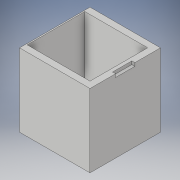
# Autodesk Inventor part: Base1
Saved by Autodesk Inventor 2017 (Build 210142000, 142)
## iProperties
Created: 2018-12-22
Part Number: Base1
Material: Generic
Document SubType Name: Modeling
Designer: Cj Lohnes
Density: 1 g/cm^3
Appearance: Default
Mass: 460.828 g
Surface Area: 957.236 cm^2
Volume: 460.828 cm^3
Author: Cj Lohnes
Autodesk Inventor part; units mm, degrees
ref_plane "YZ Plane" through (0, 0, 0) normal (1, 0, 0) x (0, 1, 0)
ref_plane "XZ Plane" through (0, 0, 0) normal (0, 1, 0) x (-1, 0, 0)
ref_plane "XY Plane" through (0, 0, 0) normal (0, 0, 1) x (1, 0, 0)
sketch "Sketch1" plane through (0, 0, 0) normal (0, 1, 0) x (-1, 0, 0)
  line L0 (66.3492, 132.9478) -> (-43.6508, 132.9478)
  line L1 (-43.6508, 132.9478) -> (-43.6508, 22.9478)
  line L2 (-43.6508, 22.9478) -> (66.3492, 22.9478)
  line L3 (66.3492, 22.9478) -> (66.3492, 132.9478)
  point P0 (0, 0)
  dimension "d0" = 110
  dimension "d1" = 110
  constraints: 8 end point, 2 parallel, 1 horizontal, 1 perpendicular
  measures "d0" distance of L2.end L0.start
  measures "d1" distance of L1.end L2.end
extrude "Main Base" add sketch "Sketch1" along normal blind 4
sketch "Sketch2" plane through (0, 4, 0) normal (0, 1, 0) x (1, 0, 0)
  circle A0 centre (-11.3492, -77.9478) radius 15
  line L0 (-66.3492, -132.9478) -> (43.6508, -132.9478) projected
  line L1 (43.6508, -132.9478) -> (43.6508, -22.9478) projected
  line L2 (-66.3492, -22.9478) -> (-66.3492, -132.9478) projected
  point P0 (0, 0)
  dimension "d4" = 30
  dimension "d14" = 55
  constraints: 1 centre point
  measures "d4" diameter of A0
  measures "d14" distance from line of L2 A0.centre
extrude "Middle Hole" cut sketch "Sketch2" against normal through all
sketch "Sketch3" plane through (0, 4, 0) normal (0, 1, 0) x (1, 0, 0)
  line L0 (43.6508, -132.9478) -> (43.6508, -22.9478) projected
  line L1 (43.6508, -22.9478) -> (-66.3492, -22.9478) projected
  line L2 (43.6508, -132.9478) -> (-66.3492, -132.9478)
  line L3 (-66.3492, -22.9478) -> (43.6508, -22.9478)
  line L4 (43.6508, -22.9478) -> (43.6508, -132.9478)
  line L5 (-66.3492, -122.9478) -> (33.6508, -122.9478)
  line L6 (33.6508, -122.9478) -> (33.6508, -32.9478)
  line L7 (33.6508, -32.9478) -> (-66.3492, -32.9478)
  line L8 (-66.3492, -132.9478) -> (-66.3492, -122.9478)
  line L9 (-66.3492, -32.9478) -> (-66.3492, -22.9478)
  point P0 (0, 0)
  dimension "d228" = 9.9
  dimension "d9" = 10
  constraints: 16 end point, 4 parallel, 2 perpendicular, 1 horizontal
  measures "d9" distance between parallel lines of L2 L5
extrude "Walls" add sketch "Sketch3" along normal blind 110
sketch "Sketch8" plane through (0, 114, 0) normal (0, 1, 0) x (1, 0, 0)
  line L0 (43.6508, -132.9478) -> (43.6508, -22.9478) projected
  line L1 (43.6508, -62.9478) -> (38.9677, -62.9478)
  line L2 (38.9677, -62.9478) -> (38.9677, -92.9478)
  line L3 (38.9677, -92.9478) -> (43.6508, -92.9478)
  line L4 (43.6508, -92.9478) -> (43.6508, -62.9478)
  line L5 (43.6508, -22.9478) -> (-66.3492, -22.9478) projected
  line L6 (-66.3492, -132.9478) -> (43.6508, -132.9478) projected
  point P0 (0, 0)
  dimension "d26" = 30
  dimension "d29" = 110
  dimension "d30" = 40
  dimension "d31" = 40
  constraints: 8 end point, 2 parallel, 1 horizontal, 1 perpendicular, 1 point on line
  measures "d26" distance of L1.end L2.end
  measures "d29" distance of L0.start L0.end
  measures "d30" distance between parallel lines of L5 L1
  measures "d31" distance between parallel lines of L6 L3
extrude "Back Notch" cut sketch "Sketch8" against normal blind 5
sketch "Sketch12" plane through (0, 4, 0) normal (0, 1, 0) x (1, 0, 0)
  circle A0 centre (-11.3492, -77.9478) radius 15 projected
  line L0 (3.6508, -77.9478) -> (-26.3492, -77.9478)
  arc A1 (-11.3492, -95.9478) -> (-11.3492, -59.9478) centre (-11.3492, -77.9478) ccw
  line L1 (-11.3492, -59.9478) -> (-11.3492, -95.9478)
  arc A2 (-11.3492, -92.9478) -> (-11.3492, -62.9478) centre (-11.3492, -77.9478) ccw
  point P0 (0, 0)
  dimension "d55" = 3
  constraints: 6 point on circle, 4 end point, 2 centre point, 2 coincident, 2 point on line, 1 concentric, 1 horizontal, 1 vertical
  measures "d55" radial gap between concentric circles of A0 A1
extrude "Extrusion10" add sketch "Sketch12" along normal blind 2.9 contours A0 L1 A1
fillet "Fillet5" radius 2 1 edges at (6.6508, 6.9, 77.9478)
sketch "Sketch11" plane through (0, 4, 0) normal (0, 1, 0) x (1, 0, 0)
  line L0 (3.6508, -77.9478) -> (3.6508, -77.9478)
  circle A0 centre (-11.3492, -47.7978) radius 4.95
  line L1 (3.6508, -77.9478) -> (-26.3492, -77.9478)
  circle A1 centre (-11.3492, -77.9478) radius 15 projected
  circle A2 centre (-11.3492, -108.0978) radius 4.95
  point P0 (0, 0)
  point P1 (-11.3492, -77.9478)
  dimension "d51" = 30.15
  dimension "d52" = 9.9
  dimension "d227" = 30.15
  dimension "d228" = 9.9
  constraints: 4 end point, 2 centre point, 1 horizontal, 1 horizontal alignment, 1 symmetric about line, 2 other
  measures "d51" distance of point (-11.349, -77.948) A0.centre
  measures "d52" diameter of A0
  measures "d227" distance from line of A2.centre L1
  measures "d228" diameter of A2
extrude "Extrusion11" add sketch "Sketch11" along normal blind 9.9 contours A0 | A2
sketch "Sketch15" plane through (0, 4, 0) normal (0, 1, 0) x (1, 0, 0)
  line L0 (-51.3492, -47.9478) -> (-46.3492, -47.9478)
  line L1 (-46.3492, -47.9478) -> (-46.3492, -57.4478)
  line L2 (-46.3492, -57.4478) -> (-51.3492, -57.4478)
  line L3 (-51.3492, -57.4478) -> (-51.3492, -47.9478)
  line L4 (-66.3492, -32.9478) -> (-66.3492, -122.9478) projected
  line L5 (-66.3492, -32.9478) -> (33.6508, -32.9478) projected
  line L6 (-23.5492, -47.9478) -> (-18.5492, -47.9478)
  line L7 (-18.5492, -47.9478) -> (-18.5492, -57.4478)
  line L8 (-18.5492, -57.4478) -> (-23.5492, -57.4478)
  line L9 (-23.5492, -57.4478) -> (-23.5492, -47.9478)
  line L10 (-21.0492, -47.9478) -> (-21.0492, -57.4478)
  line L11 (-48.8492, -47.9478) -> (-48.8492, -57.4478)
  point P0 (0, 0)
  point P1 (-59.2492, -32.9478)
  point P2 (-66.3492, -22.9478)
  point P3 (-66.3492, -132.9478)
  dimension "d71" = 9.5
  dimension "d72" = 5
  dimension "d74" = 15
  dimension "d76" = 5
  dimension "d186" = 27.8
  constraints: 20 end point, 4 midpoint, 4 parallel, 2 horizontal, 2 perpendicular
  measures "d71" distance of L2.end L0.start
  measures "d72" distance of L0.start L0.end
  measures "d74" distance from line of L5 L0.start
  measures "d76" distance of L6.start L6.end
  measures "d186" distance between parallel lines of L10 L11
extrude "Extrusion13" add sketch "Sketch15" along normal blind 23.837
fillet "Fillet6" radius 2 4 edges at (-51.3492, 27.837, 52.6978) (-46.3492, 27.837, 52.6978) (-23.5492, 27.837, 52.6978) (-18.5492, 27.837, 52.6978)
sketch "Sketch23" plane through (0, 4, 0) normal (0, 1, 0) x (1, 0, 0)
  line L0 (-11.3492, -62.4478) -> (-66.3492, -62.4478)
  line L1 (-66.3492, -62.4478) -> (-11.3492, -62.4478)
  line L2 (-66.3492, -31.5775) -> (-66.3492, -121.5775)
  line L3 (-66.3492, -62.4478) -> (-66.3492, -15.5198)
  line L4 (-11.3492, -59.9478) -> (-66.3492, -59.9478)
  line L5 (-11.3492, -59.9478) -> (-66.3492, -59.9478)
  line L6 (-66.3492, -59.9478) -> (-66.3492, -62.4478)
  line L7 (-66.3492, -62.4478) -> (-11.3492, -62.4478)
  line L8 (-11.3492, -62.4478) -> (-11.3492, -59.9478)
  line L9 (-11.3492, -95.9478) -> (-11.3492, -93.9478) projected
  line L10 (-11.3492, -95.9478) -> (-66.3492, -95.9478)
  line L11 (-66.3492, -22.9478) -> (-66.3492, -132.9478) projected
  line L12 (-66.3492, -93.4478) -> (-11.3492, -93.4478)
  line L13 (-66.3492, -93.4478) -> (-66.3492, -95.9478)
  arc A0 (-11.3492, -95.9478) -> (-11.3492, -59.9478) centre (-11.3492, -77.9478) ccw projected
  line L14 (-11.3492, -59.9478) -> (-11.3492, -93.4478)
  line L15 (-11.3492, -61.9478) -> (-11.3492, -59.9478) projected
  line L16 (-11.3492, -62.4478) -> (-11.3492, -59.9478)
  line L17 (-11.3492, -59.9478) -> (-66.3492, -59.9478)
  line L18 (-66.3492, -59.9478) -> (-11.3492, -59.9478)
  line L19 (-11.3492, -59.9478) -> (-11.3492, -62.4478)
  line L20 (-11.3492, -62.4478) -> (-66.3492, -62.4478)
  line L21 (-66.3492, -62.4478) -> (-66.3492, -59.9478)
  line L22 (-66.3492, -93.4478) -> (-11.3492, -93.4478)
  line L23 (-11.3492, -93.4478) -> (-11.3492, -95.9478)
  line L24 (-11.3492, -95.9478) -> (-66.3492, -95.9478)
  line L25 (-66.3492, -95.9478) -> (-66.3492, -93.4478)
  point P0 (0, 0)
  dimension "d216" = 2.5
  dimension "d219" = 2.5
  constraints: 46 end point, 6 parallel, 5 point on line, 4 perpendicular, 3 horizontal, 1 collinear, 1 vertical
  measures "d216" distance between parallel lines of L0 L5
  measures "d219" distance between parallel lines of L10 L12
sketch "Sketch25" plane through (-51.3492, 4, 57.4478) normal (0, 0, 1) x (1, 0, 0)
  circle A0 centre (2.388, 8.5) radius 0.9
  line L0 (0, 0) -> (0, 21.837) projected
  line L1 (32.8, 0) -> (27.8, 0) projected
  line L2 (0, 0) -> (32.8, 0)
  line L3 (16.4, 0) -> (16.4, 38.3245)
  circle A1 centre (2.388, 10.933) radius 0.9
  circle A2 centre (2.388, 13.366) radius 0.9
  circle A3 centre (2.388, 15.799) radius 0.9
  circle A4 centre (2.388, 18.232) radius 0.9
  circle A5 centre (2.388, 20.665) radius 0.9
  circle A6 centre (30.3, 8.5) radius 0.9
  circle A7 centre (30.3, 10.933) radius 0.9
  circle A8 centre (30.3, 13.366) radius 0.9
  circle A9 centre (30.3, 15.799) radius 0.9
  circle A10 centre (30.3, 18.232) radius 0.9
  circle A11 centre (30.3, 20.665) radius 0.9
  line L4 (5, 0) -> (5, 21.837) projected
  line L5 (5, 17.699) -> (27.8, 18.332)
  line L6 (27.8, 0) -> (27.8, 21.837) projected
  line L7 (29.8, 23.837) -> (30.8, 23.837) projected
  line L8 (30.3, 23.837) -> (30.3, 45.4351)
  point P0 (51.3492, -4)
  dimension "d200" = 1.8
  dimension "d201" = 8.5
  dimension "d204" = 2.433
  dimension "d207" = 27.912
  dimension "d210" = 22.8
  dimension "d211" = 11.4
  dimension "d212" = 27.912
  constraints: 12 centre point, 8 end point, 3 vertical, 2 midpoint, 2 point on line, 1 collinear, 1 horizontal, 22 other
  measures "d200" diameter of A0
  measures "d201" distance from line of L2 A0.centre
  measures "d204" distance of A0.centre A1.centre
  measures "d207" distance of A0.centre A6.centre
  measures "d210" horizontal distance of L5.start L5.end
  measures "d211" distance between parallel lines of L6 L3
  measures "d212" distance from line of L8 A5.centre
extrude "Servo Mount Holes" cut sketch "Sketch25" against normal blind 10 contours A0 | A1 | A2 | A3 | A4 | A5 | A6 | A7 | A8 | A9 | A10 | A11
extrude "Extrusion22" add sketch "Sketch23" along normal blind 3 contours L0 L2 L4 L8 | L23 L9 L10 L2 L12
fillet "Fillet7" radius 2 2 edges at (-38.8492, 7, 59.9478) (-38.8492, 7, 95.9478)
sketch "Sketch27" plane through (0, 0, 0) normal (0, -1, 0) x (1, 0, 0)
  line L0 (-54.3492, 120.9478) -> (-44.3492, 120.9478)
  line L1 (-44.3492, 120.9478) -> (-44.3492, 110.9478)
  line L2 (-44.3492, 110.9478) -> (-54.3492, 110.9478)
  line L3 (-54.3492, 110.9478) -> (-54.3492, 120.9478)
  line L4 (-66.3492, 132.9478) -> (43.6508, 132.9478) projected
  line L5 (-66.3492, 22.9478) -> (-66.3492, 132.9478) projected
  line L6 (-11.3492, 132.9478) -> (-11.3492, 22.9478)
  line L7 (43.6508, 22.9478) -> (-66.3492, 22.9478) projected
  line L8 (43.6508, 132.9478) -> (43.6508, 22.9478) projected
  line L9 (43.6508, 77.9478) -> (-66.3492, 77.9478)
  line L10 (31.6508, 120.9478) -> (21.6508, 120.9478)
  line L11 (21.6508, 120.9478) -> (21.6508, 110.9478)
  line L12 (21.6508, 110.9478) -> (31.6508, 110.9478)
  line L13 (31.6508, 110.9478) -> (31.6508, 120.9478)
  line L14 (-54.3492, 34.9478) -> (-44.3492, 34.9478)
  line L15 (-44.3492, 34.9478) -> (-44.3492, 44.9478)
  line L16 (-44.3492, 44.9478) -> (-54.3492, 44.9478)
  line L17 (-54.3492, 44.9478) -> (-54.3492, 34.9478)
  point P0 (0, 0)
  dimension "d229" = 10
  dimension "d230" = 12
  dimension "d231" = 10
  dimension "d232" = 12
  constraints: 28 end point, 8 symmetric about line, 4 midpoint, 2 parallel, 1 horizontal, 1 perpendicular
  measures "d229" distance of L0.start L0.end
  measures "d230" distance between parallel lines of L4 L0
  measures "d231" distance of L2.end L0.start
  measures "d232" distance between parallel lines of L5 L3
extrude "Extrusion24" cut sketch "Sketch27" against normal through all contours L0 L1 L2 L3 | L13 L12 L11 L10 | L17 L16 L15 L14
sketch "Sketch28" plane through (0, 4, 0) normal (0, 1, 0) x (1, 0, 0)
  line L0 (-66.3492, -22.9478) -> (-66.3492, -132.9478) projected
  line L1 (-66.3492, -132.9478) -> (43.6508, -132.9478) projected
  line L2 (-66.3492, -22.9478) -> (-64.3492, -22.9478)
  line L3 (-64.3492, -22.9478) -> (-64.3492, -132.9478)
  line L4 (-64.3492, -132.9478) -> (-66.3492, -132.9478)
  line L5 (-66.3492, -132.9478) -> (-66.3492, -22.9478)
  point P0 (0, 0)
  dimension "d237" = 2
  constraints: 8 end point, 2 parallel, 1 horizontal, 1 perpendicular, 1 point on line
  measures "d237" distance between parallel lines of L0 L3
extrude "Extrusion25" add sketch "Sketch28" along normal blind 110
equation "\"d30\" = d31"
equation "\"d76\" = d72"
body "Solid1"
